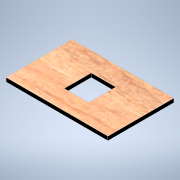
# Autodesk Inventor part: wood_front
Saved by Autodesk Inventor 2021 (Build 250183000, 183)
## iProperties
Created: 2021-08-17
Part Number: wood_front
Material: Generisch
Document SubType Name: Modeling
Designer: Tilman
Density: 1 g/cm^3
Appearance: Eloxiert - Schwarz
Author: Tilman
Autodesk Inventor part; units mm, degrees
ref_plane "YZ Plane" through (0, 0, 0) normal (1, 0, 0) x (0, 1, 0)
ref_plane "XZ Plane" through (0, 0, 0) normal (0, 1, 0) x (-1, 0, 0)
ref_plane "XY Plane" through (0, 0, 0) normal (0, 0, 1) x (1, 0, 0)
sketch "Skizze1" plane through (0, 0, 0) normal (0, 1, 0) x (-1, 0, 0)
  line L0 (0, 0) -> (-79.5, 0)
  line L1 (-79.5, 0) -> (-79.5, -51.5)
  line L2 (-79.5, -51.5) -> (0, -51.5)
  line L3 (0, -51.5) -> (0, 0)
  line L4 (-30.25, -15.25) -> (-49.25, -15.25)
  line L5 (-49.25, -15.25) -> (-49.25, -36.25)
  line L6 (-49.25, -36.25) -> (-30.25, -36.25)
  line L7 (-30.25, -36.25) -> (-30.25, -15.25)
  point P0 (-39.75, -36.25)
  point P1 (-39.75, -51.5)
  point P2 (-49.25, -25.75)
  point P3 (-79.5, -25.75)
  dimension "d0" = 79.5
  dimension "d1" = 51.5
  dimension "d4" = 21
  dimension "d5" = 19
  constraints: 16 end point, 4 midpoint, 4 parallel, 2 horizontal, 2 perpendicular, 1 horizontal alignment, 1 vertical alignment
  measures "d0" distance of L0.start L0.end
  measures "d1" distance of L2.end L0.start
  measures "d4" distance of L6.end L4.start
  measures "d5" distance of L5.end L6.end
extrude "Extrusion1" add sketch "Skizze1" along normal blind 3
